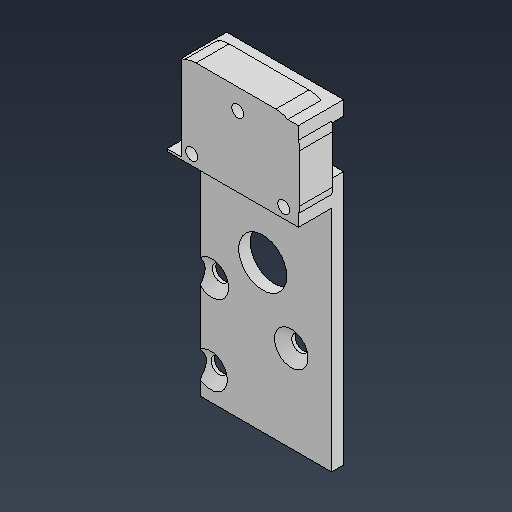
# Autodesk Inventor part: RightGearboxCover
Saved by Autodesk Inventor 2026.2 (Build 302298010, 298A)
## iProperties
Created: 2026-04-04
Part Number: RightGearboxCover
Material: Generic
Document SubType Name: Modeling
Designer: szymo
Density: 1 g/cm^3
Appearance: Default
Mass: 5.30599 g
Surface Area: 48.5829 cm^2
Volume: 5.30599 cm^3
Author: szymo
Autodesk Inventor part; units mm, degrees
ref_plane "YZ Plane" through (0, 0, 0) normal (1, 0, 0) x (0, 1, 0)
ref_plane "XZ Plane" through (0, 0, 0) normal (0, 1, 0) x (-1, 0, 0)
ref_plane "XY Plane" through (0, 0, 0) normal (0, 0, 1) x (1, 0, 0)
ref_plane "Work Plane1" through (0, -65.2958, -0.3) normal (0, 0, 1) x (1, 0, 0)
ref_plane "Work Plane4" through (0.0409, -65.2958, -0.1) normal (0, 0, 1) x (1, 0, 0)
sketch "Sketch1" plane through (0, 0, 0) normal (0, 0, 1) x (1, 0, 0)
  circle A0 centre (13, -35.9902) radius 5
  circle A1 centre (13, -35.9902) radius 5.6
  circle A2 centre (8.5216, -10.2077) radius 1.0564
  circle A3 centre (20.7784, -20.4923) radius 1.0564 construction
  circle A4 centre (14.65, -15.35) radius 5 construction
  circle A5 centre (14.65, -15.35) radius 14 construction
  circle A6 centre (14.65, -15.35) radius 14.7 construction
  circle A7 centre (14.65, -56.4236) radius 14.7 construction
  circle A8 centre (14.65, -56.4236) radius 14 construction
  line L0 (27.35, -0.65) -> (-0.05, -0.65)
  line L1 (-0.05, -0.65) -> (-0.05, -66.6236)
  line L2 (-0.05, -66.6236) -> (27.35, -66.6236)
  line L3 (27.35, -66.6236) -> (27.35, -0.65)
  line L4 (1, -17) -> (1, -13.9)
  line L5 (1, -13.9) -> (0, -13.9)
  line L6 (0, -13.9) -> (0, -18)
  line L7 (0, -18) -> (2.4477, -18)
  arc A9 (2.5, -17.9298) -> (2.4477, -18) centre (9.2084, -22.9852) ccw
  line L8 (2.5, -17.9298) -> (2.5, -17)
  line L9 (2.5, -17) -> (1, -17)
  line L10 (3, -0.65) -> (3, -18.5)
  line L11 (3, -18.5) -> (-0.05, -18.5)
  line L12 (3, -3.65) -> (27.35, -3.65)
  line L13 (27.35, -13.65) -> (3, -13.65)
  line L14 (23.6, -0.65) -> (23.6, -40.2638)
  arc A10 (20.6322, -39.1225) -> (22.0597, -39.1652) centre (21.5245, -33.1861) ccw
  arc A11 (22.0597, -39.1652) -> (22.2135, -38.6867) centre (13, -35.9902) ccw
  arc A12 (22.2135, -38.6867) -> (21.0283, -37.89) centre (18.2955, -43.2349) ccw
  arc A13 (21.0283, -37.89) -> (21.1167, -37.4672) centre (13, -35.9902) ccw
  arc A14 (21.1167, -37.4672) -> (22.5219, -37.2122) centre (20.7552, -31.475) ccw
  arc A15 (22.5219, -37.2122) -> (22.5728, -36.7122) centre (13, -35.9902) ccw
  arc A16 (22.5728, -36.7122) -> (21.2478, -36.1793) centre (19.6861, -41.9756) ccw
  arc A17 (21.2478, -36.1793) -> (21.2464, -35.7474) centre (13, -35.9902) ccw
  arc A18 (21.2464, -35.7474) -> (22.5679, -35.2058) centre (19.647, -29.9613) ccw
  arc A19 (22.5679, -35.2058) -> (22.5137, -34.7061) centre (13, -35.9902) ccw
  arc A20 (22.5137, -34.7061) -> (21.1069, -34.4603) centre (20.7844, -40.4547) ccw
  arc A21 (21.1069, -34.4603) -> (21.0157, -34.0381) centre (13, -35.9902) ccw
  arc A22 (21.0157, -34.0381) -> (22.1957, -33.2337) centre (18.2483, -28.7111) ccw
  arc A23 (22.1957, -33.2337) -> (22.0389, -32.7562) centre (13, -35.9902) ccw
  arc A24 (22.0389, -32.7562) -> (20.6117, -32.8082) centre (21.5425, -38.7387) ccw
  arc A25 (20.6117, -32.8082) -> (20.4347, -32.4142) centre (13, -35.9902) ccw
  arc A26 (20.4347, -32.4142) -> (21.4217, -31.382) centre (16.6202, -27.779) ccw
  arc A27 (21.4217, -31.382) -> (21.169, -30.9476) centre (13, -35.9902) ccw
  arc A28 (21.169, -30.9476) -> (19.7838, -31.2952) centre (21.9273, -36.9025) ccw
  arc A29 (19.7838, -31.2952) -> (19.5288, -30.9466) centre (13, -35.9902) ccw
  arc A30 (19.5288, -30.9466) -> (20.2796, -29.7317) centre (14.8338, -27.2057) ccw
  arc A31 (20.2796, -29.7317) -> (19.9421, -29.3593) centre (13, -35.9902) ccw
  arc A32 (19.9421, -29.3593) -> (18.6594, -29.9874) centre (21.9219, -35.0265) ccw
  arc A33 (18.6594, -29.9874) -> (18.3375, -29.6994) centre (13, -35.9902) ccw
  arc A34 (18.3375, -29.6994) -> (18.8193, -28.355) centre (12.9674, -27.0164) ccw
  arc A35 (18.8193, -28.355) -> (18.4117, -28.0609) centre (13, -35.9902) ccw
  arc A36 (18.4117, -28.0609) -> (17.2877, -28.9419) centre (21.5266, -33.1926) ccw
  arc A37 (17.2877, -28.9419) -> (16.9129, -28.7271) centre (13, -35.9902) ccw
  arc A38 (16.9129, -28.7271) -> (17.1047, -27.3119) centre (11.1024, -27.2193) ccw
  arc A39 (17.1047, -27.3119) -> (16.6449, -27.109) centre (13, -35.9902) ccw
  arc A40 (16.6449, -27.109) -> (15.7286, -28.2044) centre (20.7586, -31.4809) ccw
  arc A41 (15.7286, -28.2044) -> (15.3174, -28.0723) centre (13, -35.9902) ccw
  arc A42 (15.3174, -28.0723) -> (15.2107, -26.6482) centre (9.3203, -27.8055) ccw
  arc A43 (15.2107, -26.6482) -> (14.7187, -26.5453) centre (13, -35.9902) ccw
  arc A44 (14.7187, -26.5453) -> (14.0502, -27.8073) centre (19.6515, -29.9664) ccw
  arc A45 (14.0502, -27.8073) -> (13.6205, -27.7635) centre (13, -35.9902) ccw
  arc A46 (13.6205, -27.7635) -> (13.2201, -26.3927) centre (7.699, -28.7494) ccw
  arc A47 (13.2201, -26.3927) -> (12.7175, -26.3943) centre (13, -35.9902) ccw
  arc A48 (12.7175, -26.3943) -> (12.3259, -27.7677) centre (18.2538, -28.7151) ccw
  arc A49 (12.3259, -27.7677) -> (11.8965, -27.8143) centre (13, -35.9902) ccw
  arc A50 (11.8965, -27.8143) -> (11.2198, -26.5566) centre (6.3094, -30.0098) ccw
  arc A51 (11.2198, -26.5566) -> (10.7286, -26.6627) centre (13, -35.9902) ccw
  arc A52 (10.7286, -26.6627) -> (10.6311, -28.0876) centre (16.6264, -27.7817) ccw
  arc A53 (10.6311, -28.0876) -> (10.2208, -28.2224) centre (13, -35.9902) ccw
  arc A54 (10.2208, -28.2224) -> (9.2974, -27.1329) centre (5.2122, -31.5315) ccw
  arc A55 (9.2974, -27.1329) -> (8.8389, -27.3388) centre (13, -35.9902) ccw
  arc A56 (8.8389, -27.3388) -> (9.0399, -28.7528) centre (14.8405, -27.2071) ccw
  arc A57 (9.0399, -28.7528) -> (8.6665, -28.9699) centre (13, -35.9902) ccw
  arc A58 (8.6665, -28.9699) -> (7.5368, -28.0963) centre (4.4554, -33.2481) ccw
  arc A59 (7.5368, -28.0963) -> (7.1311, -28.393) centre (13, -35.9902) ccw
  arc A60 (7.1311, -28.393) -> (7.6217, -29.7343) centre (12.9742, -27.0164) ccw
  arc A61 (7.6217, -29.7343) -> (7.3016, -30.0243) centre (13, -35.9902) ccw
  arc A62 (7.3016, -30.0243) -> (6.0149, -29.4046) centre (4.072, -35.0846) ccw
  arc A63 (6.0149, -29.4046) -> (5.6799, -29.7792) centre (13, -35.9902) ccw
  arc A64 (5.6799, -29.7792) -> (6.4385, -30.9892) centre (11.109, -27.2178) ccw
  arc A65 (6.4385, -30.9892) -> (6.1858, -31.3395) centre (13, -35.9902) ccw
  arc A66 (6.1858, -31.3395) -> (4.7984, -31.0008) centre (4.0788, -36.9606) ccw
  arc A67 (4.7984, -31.0008) -> (4.5485, -31.4369) centre (13, -35.9902) ccw
  arc A68 (4.5485, -31.4369) -> (5.5422, -32.4627) centre (9.3265, -27.8027) ccw
  arc A69 (5.5422, -32.4627) -> (5.3678, -32.8578) centre (13, -35.9902) ccw
  arc A70 (5.3678, -32.8578) -> (3.9403, -32.8151) centre (4.4755, -38.7942) ccw
  arc A71 (3.9403, -32.8151) -> (3.7865, -33.2936) centre (13, -35.9902) ccw
  arc A72 (3.7865, -33.2936) -> (4.9717, -34.0903) centre (7.7045, -28.7454) ccw
  arc A73 (4.9717, -34.0903) -> (4.8833, -34.5131) centre (13, -35.9902) ccw
  arc A74 (4.8833, -34.5131) -> (3.4781, -34.7681) centre (5.2448, -40.5053) ccw
  arc A75 (3.4781, -34.7681) -> (3.4272, -35.2681) centre (13, -35.9902) ccw
  arc A76 (3.4272, -35.2681) -> (4.7522, -35.801) centre (6.3139, -30.0047) ccw
  arc A77 (4.7522, -35.801) -> (4.7536, -36.233) centre (13, -35.9902) ccw
  arc A78 (4.7536, -36.233) -> (3.4321, -36.7745) centre (6.353, -42.019) ccw
  arc A79 (3.4321, -36.7745) -> (3.4863, -37.2742) centre (13, -35.9902) ccw
  arc A80 (3.4863, -37.2742) -> (4.8931, -37.52) centre (5.2156, -31.5256) ccw
  arc A81 (4.8931, -37.52) -> (4.9843, -37.9422) centre (13, -35.9902) ccw
  arc A82 (4.9843, -37.9422) -> (3.8043, -38.7466) centre (7.7517, -43.2692) ccw
  arc A83 (3.8043, -38.7466) -> (3.9611, -39.2241) centre (13, -35.9902) ccw
  arc A84 (3.9611, -39.2241) -> (5.3883, -39.1721) centre (4.4575, -33.2416) ccw
  arc A85 (5.3883, -39.1721) -> (5.5653, -39.5661) centre (13, -35.9902) ccw
  arc A86 (5.5653, -39.5661) -> (4.5783, -40.5983) centre (9.3798, -44.2013) ccw
  arc A87 (4.5783, -40.5983) -> (4.831, -41.0328) centre (13, -35.9902) ccw
  arc A88 (4.831, -41.0328) -> (6.2162, -40.6851) centre (4.0727, -35.0778) ccw
  arc A89 (6.2162, -40.6851) -> (6.4712, -41.0337) centre (13, -35.9902) ccw
  arc A90 (6.4712, -41.0337) -> (5.7204, -42.2486) centre (11.1662, -44.7746) ccw
  arc A91 (5.7204, -42.2486) -> (6.0579, -42.621) centre (13, -35.9902) ccw
  arc A92 (6.0579, -42.621) -> (7.3406, -41.9929) centre (4.0781, -36.9538) ccw
  arc A93 (7.3406, -41.9929) -> (7.6625, -42.2809) centre (13, -35.9902) ccw
  arc A94 (7.6625, -42.2809) -> (7.1807, -43.6253) centre (13.0326, -44.9639) ccw
  arc A95 (7.1807, -43.6253) -> (7.5883, -43.9194) centre (13, -35.9902) ccw
  arc A96 (7.5883, -43.9194) -> (8.7123, -43.0384) centre (4.4734, -38.7877) ccw
  arc A97 (8.7123, -43.0384) -> (9.0871, -43.2532) centre (13, -35.9902) ccw
  arc A98 (9.0871, -43.2532) -> (8.8953, -44.6684) centre (14.8976, -44.761) ccw
  arc A99 (8.8953, -44.6684) -> (9.3551, -44.8713) centre (13, -35.9902) ccw
  arc A100 (9.3551, -44.8713) -> (10.2714, -43.7759) centre (5.2414, -40.4994) ccw
  arc A101 (10.2714, -43.7759) -> (10.6826, -43.908) centre (13, -35.9902) ccw
  arc A102 (10.6826, -43.908) -> (10.7893, -45.3321) centre (16.6797, -44.1748) ccw
  arc A103 (10.7893, -45.3321) -> (11.2813, -45.435) centre (13, -35.9902) ccw
  arc A104 (11.2813, -45.435) -> (11.9498, -44.173) centre (6.3485, -42.0139) ccw
  arc A105 (11.9498, -44.173) -> (12.3795, -44.2168) centre (13, -35.9902) ccw
  arc A106 (12.3795, -44.2168) -> (12.7799, -45.5876) centre (18.301, -43.2309) ccw
  arc A107 (12.7799, -45.5876) -> (13.2825, -45.586) centre (13, -35.9902) ccw
  arc A108 (13.2825, -45.586) -> (13.6741, -44.2126) centre (7.7462, -43.2652) ccw
  arc A109 (13.6741, -44.2126) -> (14.1035, -44.166) centre (13, -35.9902) ccw
  arc A110 (14.1035, -44.166) -> (14.7802, -45.4237) centre (19.6906, -41.9705) ccw
  arc A111 (14.7802, -45.4237) -> (15.2714, -45.3176) centre (13, -35.9902) ccw
  arc A112 (15.2714, -45.3176) -> (15.3689, -43.8927) centre (9.3736, -44.1986) ccw
  arc A113 (15.3689, -43.8927) -> (15.7792, -43.7579) centre (13, -35.9902) ccw
  arc A114 (15.7792, -43.7579) -> (16.7026, -44.8474) centre (20.7878, -40.4488) ccw
  arc A115 (16.7026, -44.8474) -> (17.1611, -44.6415) centre (13, -35.9902) ccw
  arc A116 (17.1611, -44.6415) -> (16.9601, -43.2275) centre (11.1595, -44.7732) ccw
  arc A117 (16.9601, -43.2275) -> (17.3335, -43.0104) centre (13, -35.9902) ccw
  arc A118 (17.3335, -43.0104) -> (18.4632, -43.884) centre (21.5446, -38.7322) ccw
  arc A119 (18.4632, -43.884) -> (18.8689, -43.5873) centre (13, -35.9902) ccw
  arc A120 (18.8689, -43.5873) -> (18.3783, -42.246) centre (13.0258, -44.9639) ccw
  arc A121 (18.3783, -42.246) -> (18.6984, -41.956) centre (13, -35.9902) ccw
  arc A122 (18.6984, -41.956) -> (19.9851, -42.5757) centre (21.928, -36.8957) ccw
  arc A123 (19.9851, -42.5757) -> (20.3201, -42.2011) centre (13, -35.9902) ccw
  arc A124 (20.3201, -42.2011) -> (19.5615, -40.9911) centre (14.891, -44.7625) ccw
  arc A125 (19.5615, -40.9911) -> (19.8142, -40.6409) centre (13, -35.9902) ccw
  arc A126 (19.8142, -40.6409) -> (21.2016, -40.9795) centre (21.9212, -35.0197) ccw
  arc A127 (21.2016, -40.9795) -> (21.4515, -40.5434) centre (13, -35.9902) ccw
  arc A128 (21.4515, -40.5434) -> (20.4578, -39.5176) centre (16.6735, -44.1776) ccw
  arc A129 (20.4578, -39.5176) -> (20.6322, -39.1225) centre (13, -35.9902) ccw
  circle A130 centre (13, -35.9902) radius 9.6 construction
  point P0 (0, 0)
  point P1 (23.6, -13.65)
  point P2 (23.6, -3.65)
extrude "Extrusion1" add sketch "Sketch1" against normal up to surface (0.1 mm away) contours A2 | L3 L12 L14 L0 | L14 L12 L10 L0 | L14 L13 L10 L12 | L3 L2 L1 L11 L10 L13 | A129 A128 A127 A126 A125 A124 A123 A122 A121 A120 A119 A118 A117 A116 A115 A114 A113 A112 A111 A110 A109 A108 A107 A106 A105 A104 A103 A102 A101 A100 A99 A98 A97 A96 A95 A94 A93 A92 A91 A90 A89 A88 A87 A86 A85 A84 A83 A82 A81 A80 A79 A78 A77 A76 A75 A74 A73 A72 A71 A70 A69 A68 A67 A66 A65 A64 A63 A62 A61 A60 A59 A58 A57 A56 A55 A54 A53 A52 A51 A50 A49 A48 A47 A46 A45 A44 A43 A42 A41 A40 A39 A38 A37 A36 A35 A34 A33 A32 A31 A30 A29 A28 A27 A26 A25 A24 A23 A22 A21 A20 A19 A18 A17 A16 A15 A14 A13 A12 A11 A10
ref_plane "Work Plane2" through (8.0794, -39.9218, 2.4) normal (0, 0, 1) x (0.9996763, -0.0254413, 0)
extrude "Extrusion2" add sketch "Sketch1" along normal up to surface (2.4 mm away) contours A1 | A2 | L3 L12 L14 L0 | L14 L12 L10 L0 | L14 L13 L10 L12 | L3 L2 L1 L11 L10 L13 | A129 A128 A127 A126 A125 A124 A123 A122 A121 A120 A119 A118 A117 A116 A115 A114 A113 A112 A111 A110 A109 A108 A107 A106 A105 A104 A103 A102 A101 A100 A99 A98 A97 A96 A95 A94 A93 A92 A91 A90 A89 A88 A87 A86 A85 A84 A83 A82 A81 A80 A79 A78 A77 A76 A75 A74 A73 A72 A71 A70 A69 A68 A67 A66 A65 A64 A63 A62 A61 A60 A59 A58 A57 A56 A55 A54 A53 A52 A51 A50 A49 A48 A47 A46 A45 A44 A43 A42 A41 A40 A39 A38 A37 A36 A35 A34 A33 A32 A31 A30 A29 A28 A27 A26 A25 A24 A23 A22 A21 A20 A19 A18 A17 A16 A15 A14 A13 A12 A11 A10
sketch "Sketch2" plane through (27.35, -66.6236, -0.1) normal (0, 0, -1) x (-1, 0, 0)
  circle A0 centre (12.5, 50.7958) radius 1.15 projected
  circle A1 centre (12.5, 50.7958) radius 1.65
  circle A2 centre (17.7916, 42.3106) radius 3 projected
  point P0 (27.35, 66.6236)
  dimension "d9" = 0.5
  constraints: 1 centre point
  measures "d9" radial gap between concentric circles of A0 A1
extrude "Extrusion3" cut sketch "Sketch2" against normal blind 2 contours A0 | A1
ref_plane "Work Plane3" through (1, -19, 8.2) normal (0, 0, -1) x (0, 1, 0)
ref_plane "Work Plane5" through (1, -19, 9.3) normal (0, 0, -1) x (0, 1, 0)
sketch "Sketch4" plane through (-0.05, -66.6236, 2.4) normal (0, 0, 1) x (1, 0, 0)
  circle A0 centre (14.375, 63.6236) radius 0.75 projected
  circle A1 centre (4.775, 51.0745) radius 0.75 projected
  circle A2 centre (23.975, 51.0745) radius 0.75 projected
  line L0 (23.8168, 47.6236) -> (4.9332, 47.6236) projected
  arc A3 (4.9332, 47.6236) -> (4.8944, 47.6267) centre (4.875, 47.127) ccw projected
  arc A4 (1.05, 51.6236) -> (4.8944, 47.6267) centre (5.05, 51.6236) ccw projected
  line L1 (1.05, 61.6236) -> (1.05, 51.6236) projected
  arc A5 (6.05, 66.6236) -> (1.05, 61.6236) centre (6.05, 61.6236) ccw projected
  line L2 (22.7, 66.6236) -> (6.05, 66.6236) projected
  arc A6 (27.7, 61.6236) -> (22.7, 66.6236) centre (22.7, 61.6236) ccw projected
  line L3 (27.7, 51.6236) -> (27.7, 61.6236) projected
  arc A7 (23.8556, 47.6267) -> (27.7, 51.6236) centre (23.7, 51.6236) ccw projected
  arc A8 (23.8556, 47.6267) -> (23.8168, 47.6236) centre (23.875, 47.127) ccw projected
  line L4 (23.65, 52.9736) -> (3.05, 52.9736)
  line L5 (3.05, 48.1236) -> (3.05, 65.9736) projected
  line L6 (27.4, 52.9736) -> (27.4, 0) projected
  line L7 (27.4, 47.6236) -> (0, 47.6236)
  line L8 (0, 0) -> (0, 48.1236) projected
  line L9 (23.65, 61.8736) -> (3.05, 61.8736)
  line L10 (3.05, 65.9736) -> (27.4, 65.9736) projected
  line L11 (3.05, 65.9736) -> (27.4, 65.9736) projected
  line L12 (23.65, 52.9736) -> (27.4, 52.9736) projected
  line L13 (23.65, 52.9736) -> (27.4, 52.9736) projected
  line L14 (27.4, 65.9736) -> (27.4, 62.9736) projected
  line L15 (27.4, 62.9736) -> (23.65, 62.9736) projected
  line L16 (23.65, 62.9736) -> (23.65, 52.9736) projected
  line L17 (0, 48.1236) -> (3.05, 48.1236) projected
  line L18 (3.05, 48.1236) -> (0, 48.1236)
  point P0 (0.05, 66.6236)
  point P1 (4.9332, 47.6236)
  point P2 (23.8168, 47.6236)
  point P3 (22.65, 65.2958)
  point P4 (6, 65.2958)
  point P5 (3.05, 48.1595)
  point P6 (3.05, 65.6236)
  point P7 (25.1653, 65.9736)
  point P8 (3.5847, 65.9736)
  point P9 (27.4, 63.3295)
  point P10 (4.9332, 47.6236)
  point P11 (23.8168, 47.6236)
  point P12 (27.4, 50.1038)
  point P13 (26.9651, 62.9736)
  point P14 (1.8103, 48.1236)
  dimension "d15" = 1
  constraints: 8 end point, 5 point on line, 2 horizontal, 1 collinear, 1 parallel, 1 perpendicular
  measures "d15" distance edge to line of A0 L9
extrude "Extrusion4" add sketch "Sketch4" along normal up to surface (6.9 mm away) contours A0 | A1 | A2 | L0 A3 A4 L5 L4 L12 L6 A7 A8 | A8 A7 L6 L7 | L7 L8 L17 L5 A4 A3 | L6 L12 L16 L15 L14 A6 L3 A7 | L5 L9 L16 L4 | L5 A5 L10 A6 L14 L15 L16 L9 | A6 L10 L14 | L5 L10 A5 | L10 A5 L2 A6
sketch "Sketch5" plane through (27.35, -66.6236, -0.1) normal (0, 0, -1) x (-1, 0, 0)
  circle A0 centre (12.675, 62.2958) radius 0.75 projected
  circle A1 centre (22.275, 49.7467) radius 0.75 projected
  circle A2 centre (3.075, 49.7467) radius 0.75 projected
  line L0 (3.2332, 46.2958) -> (22.1168, 46.2958) projected
  arc A3 (22.1556, 46.2989) -> (22.1168, 46.2958) centre (22.175, 45.7992) ccw projected
  arc A4 (22.1556, 46.2989) -> (26, 50.2958) centre (22, 50.2958) ccw projected
  line L1 (26, 60.2958) -> (26, 50.2958) projected
  arc A5 (26, 60.2958) -> (21, 65.2958) centre (21, 60.2958) ccw projected
  line L2 (4.35, 65.2958) -> (21, 65.2958) projected
  arc A6 (4.35, 65.2958) -> (-0.65, 60.2958) centre (4.35, 60.2958) ccw projected
  line L3 (-0.65, 50.2958) -> (-0.65, 60.2958) projected
  arc A7 (-0.65, 50.2958) -> (3.1944, 46.2989) centre (3.35, 50.2958) ccw projected
  arc A8 (3.2332, 46.2958) -> (3.1944, 46.2989) centre (3.175, 45.7992) ccw projected
  point P0 (27.35, 66.6236)
hole "Hole1" at (24.275, -16.8769, -0.1) at (14.675, -4.3278, -0.1) at (5.075, -16.8769, -0.1) direction (0, 0, 1) diameter 3 depth 4.5 counterbore diameter 3.5 counterbore depth 0.5
hole "Hole2" at (24.275, -16.8769, -0.1) at (14.675, -4.3278, -0.1) at (5.075, -16.8769, -0.1) direction (0, 0, 1) diameter 2.5 end through all
hole "Hole3" at (9.5584, -24.313, -0.1) direction (0, 0, 1) diameter 2.5 depth 2
sketch "Sketch6" plane through (-0.05, -66.6236, 2.4) normal (0, 0, 1) x (1, 0, 0)
  circle A0 centre (19.8474, 57.4238) radius 2 projected
  circle A1 centre (18.9942, 18.1118) radius 2.25 projected
  circle A2 centre (2.1786, 5.7403) radius 2 projected
  circle A3 centre (2.4496, 22.5214) radius 2 projected
  circle A4 centre (2.4496, 22.5214) radius 2.25 projected
  arc A5 (17.5031, 41.5375) -> (17.5975, 42.761) centre (19.7086, 41.9827) ccw projected
  point P0 (0.05, 66.6236)
  point P1 (19.7, 61.7958)
hole "Hole4" at (19.7974, -9.1999, 2.4) at (18.9442, -48.5119, 2.4) at (2.1286, -60.8834, 2.4) at (2.3996, -44.1023, 2.4) direction (0, 0, -1) diameter 3.4 depth 7 countersink diameter 7 countersink angle 90 clearance for "Countersunk Flat Head Screw ISO 2009/7046" size "M3" standard "ISO"
body "Solid1"
